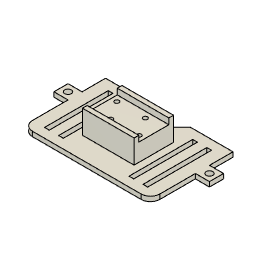
Stepper_Hood_IMU_mount_v7 (Autodesk Fusion 360 design; units mm, degrees)
Autodesk Fusion 360 part; units mm, degrees
sketch "Sketch1" plane through (0, 0, 0) normal (0, 1, 0) x (1, 0, 0)
  line L0 (0, 12.575) -> (27.15, 12.575) construction
  line L1 (27.15, 12.575) -> (27.15, -8.575)
  line L2 (23.15, -12.575) -> (0, -12.575)
  line L3 (27.15, 12.575) -> (33.15, 12.575)
  line L4 (33.15, 12.575) -> (33.15, 6.575)
  line L5 (33.15, 6.575) -> (27.15, 6.575)
  line L6 (27.15, 6.575) -> (27.15, 12.575)
  line L7 (0, -12.575) -> (0, 12.575) construction
  circle A0 centre (30.15, 9.575) radius 1.425
  line L8 (27.15, 6.575) -> (33.15, 12.575) construction
  arc A1 (23.15, -12.575) -> (27.15, -8.575) centre (23.15, -8.575) ccw
  line L9 (-27.15, 12.575) -> (-27.15, -8.575)
  line L10 (-33.15, 6.575) -> (-27.15, 6.575)
  circle A2 centre (-30.15, 9.575) radius 1.425
  line L11 (-27.15, 12.575) -> (-33.15, 12.575)
  line L12 (-33.15, 12.575) -> (-33.15, 6.575)
  line L13 (-23.15, -12.575) -> (0, -12.575)
  arc A3 (-27.15, -8.575) -> (-23.15, -12.575) centre (-23.15, -8.575) ccw
  line L14 (-27.15, 0) -> (27.15, 0) construction
  line L15 (-27.15, 12.575) -> (-27.15, 22.575)
  line L16 (-27.15, 22.575) -> (27.15, 22.575)
  line L17 (27.15, 22.575) -> (27.15, 12.575)
  line L18 (22, 18.575) -> (20, 18.575)
  line L19 (22, -8.575) -> (22, 18.575)
  line L20 (20, -8.575) -> (22, -8.575)
  line L21 (20, 18.575) -> (20, -8.575)
  line L22 (16, -8.575) -> (16, 18.575)
  line L23 (14, 18.575) -> (14, -8.575)
  line L24 (14, -8.575) -> (16, -8.575)
  line L25 (16, 18.575) -> (14, 18.575)
  line L26 (-4, 17.575) -> (4, 17.575)
  line L27 (-4, 17.575) -> (-9, 22.575)
  line L28 (4, 17.575) -> (9, 22.575)
  line L29 (11, 13.4) -> (11, -3.4)
  line L30 (-11, -3.4) -> (-11, 13.4)
  line L31 (-11, 11.4) -> (11, 11.4)
  line L32 (-11, -1.4) -> (11, -1.4)
  line L33 (-11, 13.4) -> (11, 13.4)
  line L34 (-11, -3.4) -> (11, -3.4)
  line L35 (-11, 5) -> (11, 5) construction
  line L36 (-14, -8.575) -> (-16, -8.575)
  line L37 (-14, 18.575) -> (-14, -8.575)
  line L38 (-16, -8.575) -> (-16, 18.575)
  line L39 (-16, 18.575) -> (-14, 18.575)
  line L40 (-22, 18.575) -> (-20, 18.575)
  line L41 (-20, 18.575) -> (-20, -8.575)
  line L42 (-22, -8.575) -> (-22, 18.575)
  line L43 (-20, -8.575) -> (-22, -8.575)
  circle A4 centre (3.52, 8.86) radius 0.925
  circle A5 centre (8.6, 1.14) radius 0.925
  circle A6 centre (-8.6, 8.86) radius 0.925
  circle A7 centre (-3.52, 1.14) radius 0.925
  point P0 (0, 17.575)
  point P1 (0, 5)
  dimension "d1" = 6
  dimension "d2" = 6
  dimension "d4" = 33.15
  dimension "d5" = 2.85
  dimension "d6" = 4
  dimension "d16" = 10
  dimension "d18" = 25.15
  dimension "d25" = 5
  dimension "d26" = 45
  dimension "d27" = 45
  dimension "d28" = 8
  dimension "d29" = 22
  dimension "d32" = 12.8
  dimension "d33" = 2
  dimension "d34" = 2
  dimension "d36" = 5
  dimension "d37" = 2
  dimension "d38" = 27.15
  dimension "d39" = 14
  dimension "d40" = 4
  dimension "d41" = 4
  dimension "d56" = 2.4
  dimension "d57" = 2.54
  dimension "d58" = 2.54
  dimension "d59" = 7.48
  dimension "d60" = 1.85
  dimension "d61" = 2.4
  dimension "d62" = 2.54
  dimension "d63" = 7.48
  dimension "d64" = 2.54
  constraint horizontal L0
  constraint vertical L1
  constraint horizontal L2
  constraint horizontal L3
  constraint vertical L4
  constraint horizontal L5
  constraint vertical L6
  constraint coincident L1 L0.end
  constraint perpendicular L0 L7
  constraint midpoint origin L7
  constraint collinear L0 L3
  constraint midpoint A0.centre L8
  constraint tangent L1 A1
  constraint tangent L2 A1
  constraint symmetric L0.end L7 L9.start
  constraint symmetric L2.end L7 L13.end
  constraint symmetric L3.end L7 L11.end
  constraint symmetric L4.end L7 L10.start
  constraint symmetric L5.end L7 L10.end
  constraint symmetric L7 A0 A2
  constraint symmetric L7 L1.end L9.end
  constraint symmetric L7 L2.start L13.start
  constraint symmetric L7 A1 A3
  constraint coincident L9 L14.start
  constraint coincident L1 L14.end
  constraint perpendicular L1 L14
  constraint midpoint origin L14
  constraint perpendicular L11 L15
  constraint perpendicular L15 L16
  constraint vertical L17
  constraint coincident L16 L27.end
  constraint coincident L16 L28.end
  constraint midpoint L26 P0
  constraint vertical origin P0
  constraint vertical L29
  constraint vertical L30
  constraint coincident L30 L31.start
  constraint coincident L29 L31.end
  constraint perpendicular L29 L31
  constraint coincident L30 L32.start
  constraint coincident L29 L32.end
  constraint perpendicular L29 L32
  constraint perpendicular L29 L33
  constraint horizontal L29.end L30.start
  constraint midpoint L30 L35.start
  constraint midpoint L29 L35.end
  constraint midpoint L35 P1
  constraint vertical origin P1
  constraint perpendicular L23 L24
  constraint perpendicular L22 L24
  constraint perpendicular L22 L25
  constraint equal L20 L24
  constraint equal L21 L23
  constraint perpendicular L20 L21
  constraint perpendicular L18 L19
  constraint equal L18 L25
  constraint vertical L21
  constraint horizontal L18.end L22.end
  constraint symmetric L7 L18.start L40.start
  constraint symmetric L7 L18.end L40.end
  constraint symmetric L7 L19.start L42.start
  constraint symmetric L7 L20.start L41.end
  constraint symmetric L7 L22.start L36.end
  constraint symmetric L7 L22.end L38.end
  constraint symmetric L7 L23.start L37.start
  constraint symmetric L7 L23.end L36.start
  constraint equal A4 A5
  constraint equal A6 A7
  constraint equal A4 A6
  measures "d1" distance of L3.end L4.end
  measures "d2" distance of L4 L6
  measures "d4" distance of origin L4
  measures "d5" diameter of A0
  measures "d6" radius of A1
  measures "d16" distance of L9.start L15.end
  measures "d18" distance of L0.start L2.end
  measures "d25" distance of L16 L26
  measures "d26" angle of L16 L27
  measures "d27" angle of L16 L28
  measures "d28" distance of L26.start L26.end
  measures "d29" distance of L30.end L29.start
  measures "d32" distance of L31 L32
  measures "d33" distance of L31 L33
  measures "d34" distance of L32 L34
  measures "d36" distance of origin P1
  measures "d37" distance of L22.start L23.end
  measures "d38" distance of L23.start L23.end
  measures "d39" distance of L23 P1
  measures "d40" distance of L2 L24
  measures "d41" distance of L21 L22
  measures "d56" distance of L29 A5.centre
  measures "d57" distance of L32 A5.centre
  measures "d58" distance of L31 A4.centre
  measures "d59" distance of L29 A4.centre
  measures "d60" diameter of A5
  measures "d61" distance of L30 A6.centre
  measures "d62" distance of L31 A6.centre
  measures "d63" distance of L30 A7.centre
  measures "d64" distance of L32 A7.centre
extrude "Extrude1" add sketch "Sketch1" along normal blind 2 contours L1 L3 L4 L5 L6 | L1 L2 L6 A1 L9 L13 A3 L15 L16 L17 L26 L27 L28 | L9 L10 L11 L12 | L29 L30 L31 L33 | L29 L30 L31 L32 | L29 L30 L32 L34 | A4 | A5 | A6 | A7
extrude "Extrude2" add sketch "Sketch1" along normal blind 10 from surface at 2 contours L29 L30 L31 L33 | L29 L30 L31 L32 | L29 L30 L32 L34 | A4 | A5 | A6 | A7
extrude "Extrude3" cut sketch "Sketch1" against normal blind 2.5 from surface at 12 contours L29 L30 L31 L32 | A4 | A5 | A6 | A7
extrude "Extrude4" cut sketch "Sketch1" against normal blind 8 from surface at 9.5 contours A4 | A5 | A6 | A7
